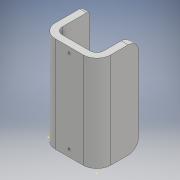
# Autodesk Inventor part: BREAD
Saved by Autodesk Inventor 2017 (Build 210142000, 142)
## iProperties
Created: 2019-09-14
Part Number: BREAD
Material: Generic
Document SubType Name: Modeling
Designer: Admin
Density: 1 g/cm^3
Appearance: Default
Mass: 229.417 g
Surface Area: 520.026 cm^2
Volume: 229.417 cm^3
Author: Admin
Autodesk Inventor part; units mm, degrees
ref_plane "YZ Plane" through (0, 0, 0) normal (1, 0, 0) x (0, 1, 0)
ref_plane "XZ Plane" through (0, 0, 0) normal (0, 1, 0) x (-1, 0, 0)
ref_plane "XY Plane" through (0, 0, 0) normal (0, 0, 1) x (1, 0, 0)
sketch "Sketch1" plane through (0, 0, 0) normal (0, 0, 1) x (1, 0, 0)
  line L0 (0, 0) -> (80, 0)
  line L1 (80, 0) -> (80, 60)
  line L2 (80, 60) -> (0, 60)
  line L3 (0, 60) -> (0, 0)
  dimension "d0" = 80
  dimension "d1" = 60
  constraints: 8 end point, 3 perpendicular, 1 horizontal
  measures "d0" distance of L0.start L0.end
  measures "d1" distance of L0.end L1.end
extrude "Extrusion1" add sketch "Sketch1" along normal blind 138
shell "Shell1" thickness 10 removed faces 3 at (53.3333, 60, 46) at (26.6667, 40, 138) at (26.6667, 40, 0)
fillet "Fillet1" radius 10 2 edges at (10, 10, 69) (70, 10, 69)
fillet "Fillet2" radius 20 1 edges at (80, 0, 69)
fillet "Fillet3" radius 20 1 edges at (0, 0, 69)
sketch "Sketch2" plane through (80, 60, 138) normal (1, 0, 0) x (0, 0, -1)
  point P0 (138, -60)
fillet "Fillet4" radius 15 1 edges at (75, 60, 0)
fillet "Fillet5" radius 15 1 edges at (75, 60, 138)
fillet "Fillet6" radius 5 1 edges at (5, 60, 138)
fillet "Fillet7" radius 5 1 edges at (5, 60, 0)
sketch "Sketch5" plane through (20, 10, 0) normal (0, 1, 0) x (1, 0, 0)
  line L0 (40, -138) -> (0, -138) projected
  line L1 (0, 0) -> (40, 0) projected
  circle A0 centre (20, -130) radius 1.5
  circle A1 centre (20, -10) radius 1.5
  point P0 (-20, 0)
  dimension "d13" = 3
  dimension "d15" = 3
  constraints: 2 centre point
  measures "d13" diameter of A0
  measures "d15" diameter of A1
extrude "Extrusion2" cut sketch "Sketch5" against normal through all
thread "Thread1" size "M3x0.5" class "6H" standard "ANSI Metric M Profile" full length
thread "Thread2" size "M3x0.5" class "6H" standard "ANSI Metric M Profile" full length
sketch "Sketch6" plane through (20, 10, 0) normal (0, 1, 0) x (1, 0, 0)
  point P0 (-20, 0)
body "Solid1"
